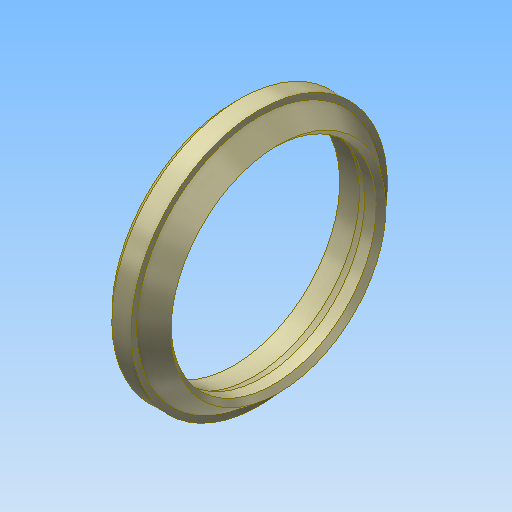
# Autodesk Inventor part: Collar_Seal_Outer
Saved by Autodesk Inventor 2020.1 (Build 241239000, 239)
## iProperties
Created: 2001-02-20
Part Number: Collar_Seal_Outer
Document SubType Name: Modeling
Designer: Joe M
Material: Nylon-6/6
Description: Wiper
Engineer: Joe M
Density: 1.13 g/cm^3
Appearance: Nylon 6
Control State: 0
Master: False
Checked Out: False
Shininess: 31.0
Length Units: 11269
Angle Units: 11279
Time Units: 11290
Mass Units: 11283
Length Display Precision: 3
Angle Display Precision: 2
Compacted: True
Density: 1.13
Volumn: 2.191563285222484
Area: 21.99018715501049
PropertySet Name: Model Information
Title: Avstrykare
Author: Joe M
Autodesk Inventor part; units mm, degrees
ref_plane "YZ Plane" through (0, 0, 0) normal (1, 0, 0) x (0, 1, 0)
ref_plane "XZ Plane" through (0, 0, 0) normal (0, 1, 0) x (-1, 0, 0)
ref_plane "XY Plane" through (0, 0, 0) normal (0, 0, 1) x (1, 0, 0)
sketch "Sketch1" plane through (0, 0, 0) normal (0, 0, 1) x (1, 0, 0)
  line L0 (4, 19.1204) -> (4, 20)
  line L1 (4, 20) -> (0, 20)
  line L2 (0, 20) -> (0, 16.5676)
  line L3 (0, 16.5676) -> (3.0669, 16.5676)
  line L4 (3.0669, 16.5676) -> (4.4257, 16)
  line L5 (4.4257, 16) -> (6.2458, 16)
  line L6 (6.2458, 16) -> (7, 16.7884)
  line L7 (7, 16.7884) -> (4, 19.1204)
  line L8 (0, 0) -> (20.4487, 0)
  dimension "d0" = 84.13
  dimension "d1" = 133.729
  dimension "d2" = 111.058
  dimension "d3" = 4
  dimension "d4" = 0.5675
  dimension "d5" = 4
  dimension "d6" = 0.7884
  dimension "d7" = 3
  dimension "d8" = 1.7197
  dimension "d9" = 32
  constraints: 18 end point, 4 parallel, 1 horizontal, 1 vertical, 1 vertical alignment
  measures "d0" angle of L7 L6
  measures "d1" angle of L6 L5
  measures "d2" angle of L6 L4
  measures "d3" distance between parallel lines of L5 L1
  measures "d4" distance between parallel lines of L5 L3
  measures "d5" distance between parallel lines of L0 L2
  measures "d6" distance from line of L6.end L5
  measures "d7" distance from line of L6.end L0
  measures "d8" distance from line of L6.end L4
  measures "d9" diameter of L5 L8
revolve "Revolution1" add sketch "Sketch1" angle 360 about axis through (0, 0, 0) along (1, 0, 0)
chamfer "Fase1" distance 1 angle 45 1 edges at (0, -20, 0)
body "Solid1"
